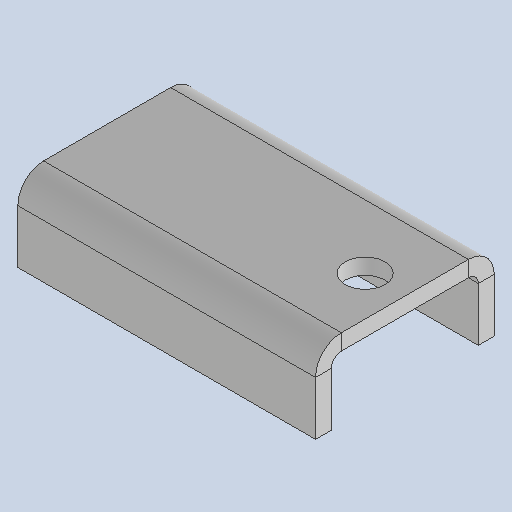
# Autodesk Inventor part: PRS 9785 leg floor channel_D1200 940
Saved by Autodesk Inventor 2026.2 (Build 302298000, 298)
## iProperties
Created: 2025-02-20
Part Number: PRS 9785 leg floor channel_D1200 940
Material: Steel
Document SubType Name: Sheet Metal
Designer: admin
Mass: 1358.18 g
Surface Area: 484.97 cm^2
Volume: 173.016 cm^3
Density: 7.85 g/cm^3
Flat Pattern Width: 14.4766 cm
Flat Pattern Length: 15 cm
Flat Pattern Area: 217.15 cm^2
Sheet Metal Rule: AISI304 3mm Die 32
Sheet Metal Width: 144,766 mm
Sheet Metal Length: 150,000 mm
Sheet Metal Area: 21714,955 mm^2
Appearance: Default
Author: user
Autodesk Inventor part; units mm, degrees
ref_plane "YZ Plane" through (0, 0, 0) normal (1, 0, 0) x (0, 1, 0)
ref_plane "XZ Plane" through (0, 0, 0) normal (0, 1, 0) x (-1, 0, 0)
ref_plane "XY Plane" through (0, 0, 0) normal (0, 0, 1) x (1, 0, 0)
sketch "Sketch1" plane through (0, 0, 0) normal (0, 0, 1) x (1, 0, 0)
  line L0 (-75, -45) -> (75, -45)
  line L1 (75, -45) -> (75, 45)
  line L2 (75, 45) -> (-75, 45)
  line L3 (-75, 45) -> (-75, -45)
  line L4 (-75, -45) -> (75, 45) construction
  line L5 (75, -45) -> (-75, 45) construction
  circle A0 centre (55, -25) radius 10
  circle A1 centre (55, 25) radius 10
  line L6 (0, 0) -> (75, 0) construction
  circle A2 centre (55, 0) radius 10
  dimension "d0" = 150
  dimension "d1" = 90
  dimension "d23" = 20
  dimension "d25" = 20
  dimension "d26" = 20
  measures "d0" distance of L2.end L1.end
  measures "d1" distance of L1.end L0.end
  measures "d23" diameter of A0
  measures "d25" distance from line of L1 A0.centre
  measures "d26" distance from line of A0.centre L0
extrude "Plate1" add sketch "Sketch1" along normal blind 8 contours L3 L2 L1 L0 | A0 | A1
sketch "Sketch6" plane through (-75, -37, 8) normal (0, -1, 0) x (1, 0, 0)
  line L0 (150, 0) -> (0, 0)
  line L1 (0, 0) -> (0, -40)
  line L2 (0, -40) -> (150, -40)
  line L3 (150, -40) -> (150, 0)
  constraints: 6 end point, 1 horizontal, 1 perpendicular, 1 vertical
edge flange "Flange2" height 40 angle 90 thickness 8 bend radius 5 thickness toward (0, -1, 0) relief round relief width 8 relief depth 4 corner gap 5 corner form 0 edges at (0, -45, 0) (0, 45, 0) wall of the first edge with corners at (75, -37, 8) (-75, -37, 8) (-75, -37, -32) (75, -37, -32)
bend "Bend2"
corner "Corner2"
equation "\"d26\" = d25"
equation "\"d2\" = Thickness"
equation "\"d30\" = BendReliefWidth"
equation "\"d31\" = BendReliefDepth"
equation "\"d32\" = MinimumRemnant"
equation "\"d33\" = TransitionRadius"
equation "\"d36\" = BendRadius"
equation "\"d37\" = CornerReliefSize"
equation "\"d38\" = GapSize"
equation "\"d39\" = JacobiRadiusSize"
equation "\"BendReliefWidth\" = Thickness"
equation "\"BendReliefDepth\" = 0.5 * Thickness"
equation "\"CornerReliefSize\" = 4 * Thickness"
equation "\"MinimumRemnant\" = 2 * Thickness"
equation "\"TransitionRadius\" = BendRadius"
equation "\"JacobiRadiusSize\" = BendRadius"
equation "\"GapSize\" = Thickness"
equation "\"Thickness\" = 8"
equation "\"BendRadius\" = 5"
body "Solid1"
